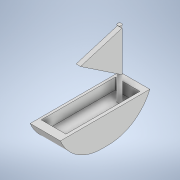
# Autodesk Inventor part: Part1
Saved by Autodesk Inventor 2021 (Build 250183000, 183)
## iProperties
Created: 2022-03-08
Part Number: Part1
Material: Generic
Document SubType Name: Sheet Metal
Designer: User
Density: 1 g/cm^3
Sheet Metal Rule: Default_mm
Appearance: Default
Author: User
Autodesk Inventor part; units mm, degrees
ref_plane "YZ Plane" through (0, 0, 0) normal (1, 0, 0) x (0, 1, 0)
ref_plane "XZ Plane" through (0, 0, 0) normal (0, 1, 0) x (-1, 0, 0)
ref_plane "XY Plane" through (0, 0, 0) normal (0, 0, 1) x (1, 0, 0)
sketch "Sketch1" plane through (0, 0, 0) normal (0, 0, 1) x (1, 0, 0)
  line L0 (-0.7644, 0.5337) -> (0.5866, 0.5337)
  line L1 (0.5866, 0.5337) -> (0.5866, -0.6988)
  line L2 (0.5866, -0.6988) -> (-0.7644, -0.6988)
  line L3 (-0.7644, -0.6988) -> (-0.7644, 0.5337)
  point P0 (0, 0)
  constraints: 8 end point, 2 parallel, 1 horizontal, 1 perpendicular
extrude "Extrusion1" add sketch "Sketch1" along normal blind 4
fillet "Fillet1" radius 2 1 edges at (-0.0889, -0.6988, 4)
fillet "Fillet2" radius 2 1 edges at (-0.0889, -0.6988, 0)
sketch "Sketch2" plane through (-0.7644, 0.5337, 4) normal (0, 1, 0) x (1, 0, 0)
  line L0 (1.2126, 0.3861) -> (0.1067, 0.3861)
  line L1 (0.1067, 0.3861) -> (0.1067, 3.6976)
  line L2 (0.1067, 3.6976) -> (1.2126, 3.6976)
  line L3 (1.2126, 3.6976) -> (1.2126, 0.3861)
  point P0 (0.7644, 4)
  constraints: 8 end point, 2 parallel, 1 horizontal, 1 perpendicular
extrude "Extrusion2" cut sketch "Sketch2" against normal blind 0.5
sketch "Sketch3" plane through (-0.7644, 0.0337, 4) normal (0, 1, 0) x (1, 0, 0)
  circle A0 centre (0.6659, 3.3334) radius 0.0901
  point P0 (0.7644, 4)
  constraints: 1 centre point
extrude "Extrusion3" add sketch "Sketch3" along normal blind 3
sketch "Sketch4" plane through (0, 0, 0) normal (1, 0, 0) x (0, 1, 0)
  line L0 (0.0337, 0.7568) -> (3.0337, 0.7568) projected
  line L1 (3.0337, 0.7568) -> (2.4774, 2.611)
  line L2 (2.4774, 2.611) -> (1.2341, 0.7568)
  line L3 (3.0337, 0.7568) -> (1.2341, 0.7568)
  point P0 (0, 0)
  constraints: 6 end point, 2 point on line, 1 collinear
extrude "Extrusion4" add sketch "Sketch4" along normal mid plane 0.2
equation "\"BendRadius\" = Thickness"
equation "\"BendReliefWidth\" = Thickness"
equation "\"BendReliefDepth\" = 0.5 * Thickness"
equation "\"CornerReliefSize\" = 4 * Thickness"
equation "\"MinimumRemnant\" = 2 * Thickness"
equation "\"TransitionRadius\" = BendRadius"
equation "\"JacobiRadiusSize\" = BendRadius"
equation "\"GapSize\" = Thickness"
equation "\"Thickness\" = 0.5"
body "Solid1"
